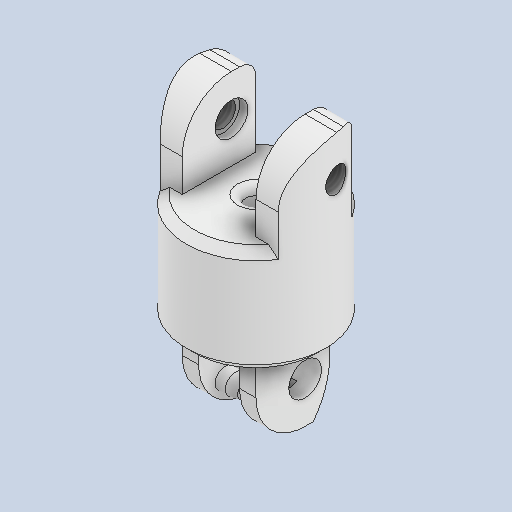
# Autodesk Inventor part: Middle_2
Saved by Autodesk Inventor 2022 (Build 260153000, 153)
## iProperties
Created: 2023-01-15
Part Number: Middle_2
Material: ABS Plastic
Document SubType Name: Modeling
Designer: 48735
Density: 1.06 g/cm^3
Appearance: Smooth - White
Author: 48735
Autodesk Inventor part; units mm, degrees
ref_plane "YZ Plane" through (0, 0, 0) normal (1, 0, 0) x (0, 1, 0)
ref_plane "XZ Plane" through (0, 0, 0) normal (0, 1, 0) x (-1, 0, 0)
ref_plane "XY Plane" through (0, 0, 0) normal (0, 0, 1) x (1, 0, 0)
sketch "Sketch1" plane through (0, 0, 0) normal (0, 1, 0) x (-1, 0, 0)
  circle A0 centre (0, 0) radius 8.5
  line L0 (0, 0) -> (-2.5, 0)
  line L1 (-2.5, 0) -> (4.5, 0)
  line L2 (4.5, 0) -> (4.5, -2.5)
  line L3 (4.5, -2.5) -> (4.5, 4.5)
  line L4 (-4.5, 0) -> (-4.5, -2.5)
  line L5 (-4.5, 4.5) -> (-4.5, 0)
  line L6 (4.5, -4.5) -> (-4.5, -4.5)
  line L7 (-2.5, -2.5) -> (2.5, -2.5)
  line L8 (-2.5, -2.5) -> (-2.5, 4.5)
  line L9 (-2.5, 4.5) -> (-4.5, 4.5)
  line L10 (2.5, -2.5) -> (2.5, 4.5)
  line L11 (2.5, 4.5) -> (4.5, 4.5)
  line L12 (-4.5, -2.5) -> (-4.5, -4.5)
  line L13 (4.5, -4.5) -> (4.5, -2.5)
  point P0 (6.5, 0)
  constraints: 28 end point, 6 point on line, 5 perpendicular, 3 vertical, 2 horizontal, 1 centre point, 1 coincident, 1 collinear
extrude "Extrusion1" add sketch "Sketch1" along normal blind 10 contours L8 L7 L10 L1 L2 L13 L6 L12 L4 L5 L9 | L10 L11 L3 L1
sketch "Sketch2" plane through (0, 10, 0) normal (0, 1, 0) x (1, 0, 0)
  circle A0 centre (0, 0) radius 8.5
  circle A1 centre (0, 0) radius 1.25
  dimension "d11" = 17
  dimension "d12" = 2.5
  constraints: 2 centre point, 2 coincident
  measures "d11" diameter of A0
  measures "d12" diameter of A1
extrude "Extrusion2" add sketch "Sketch2" along normal blind 1
fillet "Fillet4" radius 1 1 edges at (-1.25, 10, 0)
fillet "Fillet5" radius 6 2 edges at (3.5, 0, 4.5) (-3.5, 0, 4.5)
fillet "Fillet6" radius 10 1 edges at (0, 0, -4.5)
sketch "Sketch3" plane through (-4.5, 10, -4.5) normal (-1, 0, 0) x (0, 0, 1)
  arc A0 (3, -10) -> (9, -4) centre (3, -4) ccw projected
  line L0 (3, -10) -> (3, -5)
  point P0 (4.5, -10)
  dimension "d24" = 5
  constraints: 2 end point, 1 vertical
  measures "d24" distance of L0.start L0.end
hole "Hole1" at (-4.5, 5, -1.5) direction (1, 0, 0) diameter 4 depth 10
sketch "Sketch4" plane through (2.5, 10, -2.5) normal (-1, 0, 0) x (0, 0, 1)
  line L0 (7, -4) -> (7, 0) projected
  circle A0 centre (3.75, -7) radius 1.25
  point P0 (2.5, -10)
  constraints: 1 centre point
extrude "Extrusion3" add sketch "Sketch4" along normal blind 2.5
chamfer "Chamfer1" distance 0.25 distance2 1.25 1 edges at (0, 3, 0) measured on face at (0, 2.3808, 1.5915)
sketch "Sketch5" plane through (-2.5, 10, 4.5) normal (1, 0, 0) x (0, 0, -1)
  circle A0 centre (3.25, -7) radius 1.25 projected
  circle A1 centre (3.25, -7) radius 1.25
  point P0 (4.5, -10)
  constraints: 1 centre point, 1 coincident
extrude "Extrusion4" add sketch "Sketch5" along normal blind 2.5
chamfer "Chamfer2" distance 0.25 distance2 1.25 1 edges at (0, 3, 2.5) measured on face at (0, 2.8205, 0.1051)
sketch "Sketch6" plane through (0, 11, 0) normal (0, 1, 0) x (1, 0, 0)
  circle A0 centre (0, 0) radius 1.25
  circle A1 centre (0, 0) radius 8.5
  constraints: 2 centre point, 2 coincident
extrude "Extrusion5" add sketch "Sketch6" along normal blind 11
sketch "Sketch7" plane through (0, 22, 0) normal (0, 1, 0) x (1, 0, 0)
  circle A0 centre (0, 0) radius 8.5
  circle A1 centre (0, 0) radius 1.25
  dimension "d49" = 17
  dimension "d48" = 2.5
  constraints: 2 centre point, 2 coincident
  measures "d49" diameter of A0
  measures "d48" diameter of A1
extrude "Extrusion6" add sketch "Sketch7" along normal blind 1
sketch "Sketch8" plane through (0, 23, 0) normal (0, 1, 0) x (1, 0, 0)
  circle A0 centre (0, 0) radius 2.25
  circle A1 centre (0, 0) radius 8.5
  circle A2 centre (0, 0) radius 1.25
  line L0 (4.5, 0) -> (4.5, 4.5)
  line L1 (4.5, 4.5) -> (7.2111, 4.5)
  line L2 (4.5, -4.5) -> (4.5, 1.5)
  line L3 (4.5, 0) -> (4.5, -4.5)
  line L4 (7.2111, -4.5) -> (4.5, -4.5)
  line L5 (4.5, -4.5) -> (7.2111, -4.5)
  line L6 (-7.2111, 4.5) -> (-4.5, 4.5)
  line L7 (-4.5, 0) -> (-4.5, 4.5)
  line L8 (-4.5, 4.5) -> (-7.2111, 4.5)
  line L9 (-4.5, 0) -> (-4.5, -4.5)
  line L10 (-4.5, 1.5) -> (-4.5, -4.5)
  line L11 (-4.5, -4.5) -> (-7.2111, -4.5)
  point P0 (-7.2111, -4.5)
  point P1 (-7.2111, -4.5)
  constraints: 24 end point, 3 centre point, 2 point on circle, 1 coincident, 1 perpendicular, 1 vertical
extrude "Extrusion7" add sketch "Sketch8" along normal blind 10 contours A1 L4 L2 L0 L1 | L6 L7 L9 L11 A1
fillet "Fillet8" radius 6 2 edges at (-5.8556, 33, 4.5) (5.8556, 33, 4.5)
fillet "Fillet9" radius 2 2 edges at (5.8556, 33, -4.5) (-5.8556, 33, -4.5)
chamfer "Chamfer3" distance 1 angle 45 1 edges at (-8.5, 10, 0)
sketch "Sketch9" plane through (4.5, 23, -4.5) normal (-1, 0, 0) x (0, 0, 1)
  arc A0 (9, 4) -> (3, 10) centre (3, 4) ccw projected
  line L0 (3, 10) -> (3, 5)
  point P0 (4.5, -23)
  dimension "d62" = 5
  constraints: 2 end point, 1 vertical
  measures "d62" distance of L0.start L0.end
hole "Hole2" at (4.5, 28, -1.5) direction (1, 0, 0) diameter 3 depth 5 counterbore diameter 4 counterbore depth 1
sketch "Sketch10" plane through (-4.5, 23, 4.5) normal (1, 0, 0) x (0, 0, -1)
  line L0 (6, 10) -> (6, 5)
  point P0 (4.5, -23)
  dimension "d70" = 5
  constraints: 2 end point, 1 vertical
  measures "d70" distance of L0.start L0.end
hole "Hole3" at (-4.5, 28, -1.5) direction (-1, 0, 0) diameter 3 depth 5 counterbore diameter 4 counterbore depth 1
chamfer "Chamfer4" distance 1 angle 45 2 edges at (0, 23, 8.5) (0, 23, -8.5)
fillet "Fillet10" radius 1 1 edges at (-1.25, 23, 0)
thread "Thread1" size "M3x0.5" class "6H" standard "ANSI Metric M Profile" length 6
thread "Thread2" size "M3x0.5" class "6H" standard "ANSI Metric M Profile" length 6
body "Solid1"
